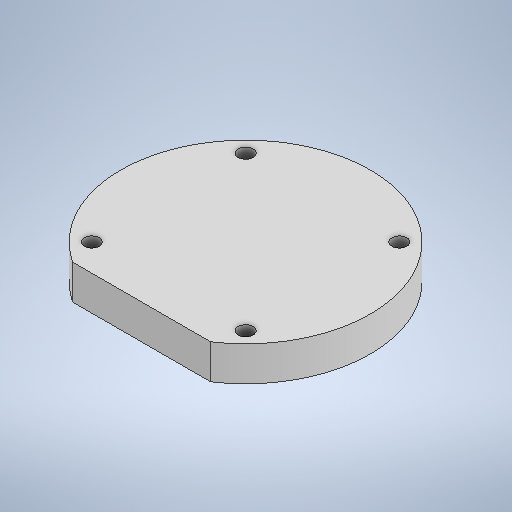
# Autodesk Inventor part: Access Cap
Saved by Autodesk Inventor 2025 (Build 290162000, 162)
## iProperties
Created: 2025-10-23
Part Number: Access Cap
Material: Generic
Document SubType Name: Modeling
Designer: mumin
Density: 1 g/cm^3
Appearance: Default
Author: mumin
Autodesk Inventor part; units mm, degrees
ref_plane "YZ Plane" through (0, 0, 0) normal (1, 0, 0) x (0, 1, 0)
ref_plane "XZ Plane" through (0, 0, 0) normal (0, 1, 0) x (-1, 0, 0)
ref_plane "XY Plane" through (0, 0, 0) normal (0, 0, 1) x (1, 0, 0)
sketch "Sketch1" plane through (0, 0, 0) normal (0, 1, 0) x (-1, 0, 0)
  circle A0 centre (0, 0) radius 36
  line L0 (19.8997, 30) -> (-19.8997, 30)
  dimension "d0" = 72
  dimension "d1" = 30
  constraints: 2 end point, 2 point on circle, 1 centre point, 1 coincident, 1 horizontal
  measures "d0" diameter of A0
  measures "d1" distance from line of point (0, 0) L0
extrude "Base" add sketch "Sketch1" along normal blind 10 contours A0 L0 picked at (-0.4083, 8.0069)
sketch "Sketch2" plane through (0, 0, 0) normal (0, -1, 0) x (1, 0, 0)
  circle A0 centre (0, 0) radius 31.4
  line L0 (22.2032, 22.2032) -> (0, 0)
  line L1 (-50.4, 0) -> (50.4, 0) projected
  dimension "d11" = 62.8
  dimension "d12" = 45
  constraints: 2 end point, 1 coincident, 3 other
  measures "d12" angle of L1 L0
hole "Mounting Holes" at (22.2032, 0, 22.2032) direction (0, 1, 0) diameter 4.3 end through all counterbore diameter 8 counterbore depth 4
pattern_circular "Circular Pattern1" count 4 over 360 about axis through (0, 0, 0) along (0, 1, 0) of "Mounting Holes"
body "Solid1"
